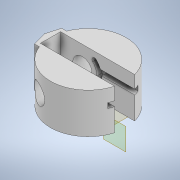
# Autodesk Inventor part: handle_base
Saved by Autodesk Inventor 2021 (Build 250183000, 183)
## iProperties
Created: 2021-03-06
Part Number: handle_base
Material: Generic
Document SubType Name: Modeling
Designer: ben
Density: 1 g/cm^3
Appearance: Default
Mass: 226.368 g
Surface Area: 425.082 cm^2
Volume: 226.368 cm^3
Author: ben
Autodesk Inventor part; units mm, degrees
ref_plane "YZ Plane" through (0, 0, 0) normal (1, 0, 0) x (0, 1, 0)
ref_plane "XZ Plane" through (0, 0, 0) normal (0, 1, 0) x (-1, 0, 0)
ref_plane "XY Plane" through (0, 0, 0) normal (0, 0, 1) x (1, 0, 0)
ref_plane "Work Plane1" through (-35, 22.5, -35) normal (0, 0, 1) x (1, 0, 0)
sketch "Sketch1" plane through (-35, 22.5, -35) normal (0, 0, 1) x (1, 0, 0)
  circle A0 centre (35, -42) radius 27.25
  circle A1 centre (35, -42) radius 6
  circle A2 centre (19, -42) radius 6
  dimension "d0" = 54.5
  dimension "d24" = 12
  dimension "d70" = 12
  dimension "d71" = 16
  constraints: 3 centre point, 1 coincident, 1 horizontal alignment, 1 other
  measures "d0" diameter of A0
  measures "d24" diameter of A1
  measures "d70" diameter of A2
  measures "d71" distance of A2.centre A0.centre
ref_plane "Work Plane2" through (0, -19.5, 0) normal (0, 0, 1) x (1, 0, 0)
sketch "Sketch2" plane through (0, -19.5, 0) normal (0, 0, 1) x (1, 0, 0)
  arc A0 (-36.1421, -10) -> (-36.1421, 10) centre (0, 0) ccw
  line L0 (37.5, -10) -> (-36.1421, -10)
  line L1 (-36.1421, 10) -> (37.5, 10)
  line L2 (37.5, 10) -> (37.5, -10)
  line L3 (34.9857, -13.5) -> (39.9857, -13.5)
  line L4 (39.9857, -13.5) -> (39.9857, 13.5)
  line L5 (39.9857, 13.5) -> (34.9857, 13.5)
  line L6 (34.9857, 13.5) -> (34.9857, -13.5)
  line L7 (39.9857, -13.5) -> (43.6938, 0)
  line L8 (43.6938, 0) -> (39.9857, 13.5)
  point P0 (0, 19.5)
  point P1 (37.5, 0)
  point P2 (36.1421, 10)
  point P3 (36.1421, -10)
  dimension "d3" = 75
  dimension "d40" = 5
  dimension "d41" = 27
  dimension "d44" = 14
  constraints: 18 end point, 4 horizontal, 4 point on circle, 3 parallel, 1 centre point, 1 perpendicular, 1 tangent, 1 vertical, 1 other
  measures "d3" diameter of A0
  measures "d40" distance of L3.start L3.end
  measures "d41" distance of L5.end L3.start
  measures "d44" distance of L3.end L7.end
extrude "Extrusion2" add sketch "Sketch2" along normal blind 40 contours L0 L6 A0 | L6 L0 A0 | A0 L0 L2 L1 L5 L4 L3 | L4 L8 L7 | L6 A0 L1 | L1 A0 L6
ref_plane "Work Plane3" through (-36.1421, -9.5, 0) normal (0, -1, 0) x (1, 0, 0)
sketch "Sketch4" plane through (-36.1421, -9.5, 0) normal (0, -1, 0) x (1, 0, 0)
  line L0 (0, 0) -> (10.5247, 0) projected
  point P0 (36.1421, 0)
  point P1 (51.9367, 20)
hole "Hole2" at (15.7946, -9.5, 20) direction (0, 1, 0) diameter 19.05 end through all both
extrude "Extrusion3" add sketch "Sketch1" along normal blind 35 and the other way blind 10
sketch "Sketch8" plane through (0, -19.5, -45) normal (0, 0, -1) x (-1, 0, 0)
  circle A0 centre (0, 0) radius 6 projected
  circle A1 centre (0, 0) radius 6 projected
  line L0 (-6, 10.3923) -> (12, 0)
  line L1 (12, 0) -> (-6, -10.3923)
  line L2 (-6, -10.3923) -> (-6, 10.3923)
  line L3 (-8, -13.8564) -> (16, 0)
  line L4 (16, 0) -> (-8, 13.8564)
  line L5 (-8, 13.8564) -> (-8, -13.8564)
  point P0 (0, 19.5)
  point P1 (-6, 0)
  point P2 (-6, 0)
  point P3 (3, -5.1962)
  point P4 (3, 5.1962)
  dimension "d69" = 2
  constraints: 12 end point, 1 coincident, 1 horizontal alignment, 1 midpoint, 10 other
  measures "d69" distance between parallel lines of L1 L3
extrude "Extrusion5" add sketch "Sketch8" along normal blind 15 contours A0 L0 L1 | A0 L2 L0 | L1 L2 A0 | L5 L4 L3
ref_plane "Work Plane4" through (-35, 22.5, 0) normal (0, 0, 1) x (1, 0, 0)
split body "Split1" result two bodies by plane through (-35, 22.5, 0) normal (0, 0, 1) first body at (28.9114, 3.5897, 20.1633)
sketch "Sketch11" plane through (0, -19.5, -45) normal (0, 0, -1) x (-1, 0, 0)
  arc A0 (10.8038, -3) -> (10.8038, 3) centre (16, 0) ccw projected
  arc A1 (10.8038, 3) -> (10.8038, -3) centre (16, 0) ccw projected
extrude "Extrusion8" add sketch "Sketch11" against normal blind 10 bodies 3
sketch "Sketch13" plane through (-36.1421, -29.5, 0) normal (0, 1, 0) x (1, 0, 0)
  line L0 (40, -20) -> (40, -20)
  circle A0 centre (51.9367, -20) radius 9.525 projected
  line L1 (0, 0) -> (0, -40) projected
  line L2 (0, -22.5) -> (32.6611, -22.5)
  arc A1 (37.4997, -20) -> (41.7282, -30.2085) centre (51.9367, -20) ccw
  line L3 (51.9367, -20) -> (41.7282, -30.2085) construction
  line L4 (51.9367, -20) -> (37.4997, -20) construction
  arc A2 (38.1927, -33.744) -> (41.7282, -30.2085) centre (39.9604, -31.9763) ccw
  arc A3 (0, -22.5) -> (0, -27.5) centre (0, -25) ccw
  line L5 (0, -27.5) -> (34.005, -27.5)
  arc A4 (32.4997, -20) -> (32.6611, -22.5) centre (51.9367, -20) ccw
  arc A5 (34.005, -27.5) -> (38.1927, -33.744) centre (51.9367, -20) ccw
  arc A6 (37.4997, -20) -> (32.4997, -20) centre (34.9997, -20) ccw
  point P0 (36.1421, 0)
  dimension "d62" = 45
  dimension "d82" = 14.437
  dimension "d83" = 5
  dimension "d84" = 45
  dimension "d85" = 2.5
  dimension "d86" = 2.5
  constraints: 13 point on circle, 10 end point, 6 centre point, 2 point on line, 2 tangent, 1 coincident, 1 equal radius, 1 horizontal
  measures "d62" angle of L4 L3
  measures "d82" distance of L4.end A0.centre
  measures "d83" radial gap between concentric circles of A5 A1
  measures "d85" radius of A3
  measures "d86" radius of A6
extrude "Extrusion9" cut sketch "Sketch13" along normal blind 25 and the other way blind 5 contours L2 A4 A6 A1 A2 A5 L5 L1 | L1 A3 bodies 2
sketch "top-bottom notch" plane through (0, -19.5, 0) normal (0, 0, 1) x (1, 0, 0)
  arc A0 (-10, -10) -> (10, -10) centre (0, -10) ccw
  line L0 (0, -10) -> (-10, -10) construction
  line L1 (0, -10) -> (10, -10) construction
  line L2 (37.5, -10) -> (-36.1421, -10) projected
  line L3 (-36.1421, 10) -> (37.5, 10) projected
  arc A1 (10, 10) -> (-10, 10) centre (0, 10) ccw
  line L4 (0, 10) -> (-10, 10) construction
  line L5 (0, 10) -> (10, 10) construction
  arc A2 (-9.4868, -10.5) -> (9.4868, -10.5) centre (0, -10) ccw
  line L6 (-9.4868, -10.5) -> (0, -10.5)
  line L7 (0, -10.5) -> (9.4868, -10.5)
  arc A3 (9.4868, 10.5) -> (-9.4868, 10.5) centre (0, 10) ccw
  line L8 (9.4868, 10.5) -> (0, 10.5)
  line L9 (0, 10.5) -> (-9.4868, 10.5)
  dimension "d87" = 10
  dimension "d88" = 180
  dimension "d89" = 10
  dimension "d90" = 180
  dimension "d91" = 0.5
  dimension "d92" = 0.5
  constraints: 16 end point, 8 point on circle, 4 centre point, 3 point on line, 4 other
  measures "d87" radius of A0
  measures "d88" angle of L1 L0
  measures "d89" radius of A1
  measures "d90" angle of L4 L5
  measures "d91" radial gap between concentric circles of A0 A2
  measures "d92" radial gap between concentric circles of A1 A3
extrude "Extrusion10" add sketch "top-bottom notch" against normal blind 5 contours L6 L7 A2 | L8 L9 A3 bodies 2
